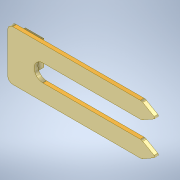
# Autodesk Inventor part: sensorhumedad
Saved by Autodesk Inventor 2022 (Build 260153000, 153)
## iProperties
Created: 2021-10-13
Part Number: sensorhumedad
Material: Brass, Soft Yellow
Document SubType Name: Modeling
Designer: pa.mahecha
Density: 8.47 g/cm^3
Appearance: Gold - Metal
Author: pa.mahecha
Autodesk Inventor part; units mm, degrees
ref_plane "YZ Plane" through (0, 0, 0) normal (1, 0, 0) x (0, 1, 0)
ref_plane "XZ Plane" through (0, 0, 0) normal (0, 1, 0) x (-1, 0, 0)
ref_plane "XY Plane" through (0, 0, 0) normal (0, 0, 1) x (1, 0, 0)
sketch "Sketch1" plane through (0, 0, 0) normal (0, 0, 1) x (1, 0, 0)
  line L0 (-9.4004, -0.0645) -> (24.8301, -0.0645)
  line L1 (-8.5062, -0.0645) -> (-8.5062, 8.0815)
  line L2 (-6.5062, 10.0815) -> (45.2045, 10.0815)
  line L3 (5.7396, 3.4575) -> (45.196, 3.4575)
  line L4 (-8.5062, -0.0645) -> (-8.5062, -8.2105)
  line L5 (-6.5062, -10.2105) -> (45.2045, -10.2105)
  line L6 (5.7396, -3.5865) -> (45.196, -3.5865)
  line L7 (50.7891, 7.186) -> (46.1991, 9.8167)
  line L8 (50.7862, 6.3168) -> (46.1793, 3.7159)
  line L9 (50.7891, -7.315) -> (46.1991, -9.9457)
  line L10 (50.7862, -6.4458) -> (46.1793, -3.8449)
  arc A0 (5.7396, 3.4575) -> (5.7396, -3.5865) centre (5.7054, -0.0645) ccw
  arc A1 (-6.5062, 10.0815) -> (-8.5062, 8.0815) centre (-6.5062, 8.0815) ccw
  arc A2 (-8.5062, -8.2105) -> (-6.5062, -10.2105) centre (-6.5062, -8.2105) ccw
  arc A3 (46.1991, 9.8167) -> (45.2045, 10.0815) centre (45.2045, 8.0815) ccw
  arc A4 (45.196, 3.4575) -> (46.1793, 3.7159) centre (45.196, 5.4575) ccw
  arc A5 (50.7862, 6.3168) -> (50.7891, 7.186) centre (50.5404, 6.7522) ccw
  line L11 (50.7891, -7.315) -> (46.1991, -9.9457)
  line L12 (50.7862, -6.4458) -> (46.1793, -3.8449)
  arc A6 (45.2045, -10.2105) -> (46.1991, -9.9457) centre (45.2045, -8.2105) ccw
  arc A7 (46.1793, -3.8449) -> (45.196, -3.5865) centre (45.196, -5.5865) ccw
  arc A8 (50.7891, -7.315) -> (50.7862, -6.4458) centre (50.5404, -6.8812) ccw
  line L13 (5.7396, 3.4575) -> (5.7396, 10.0815)
  line L14 (5.7396, -3.5865) -> (5.7396, -10.2105)
  point P0 (0, 0)
  point P1 (51.4938, 10.0604)
  point P2 (51.4938, -10.1894)
  dimension "d7" = 6.624
  dimension "d11" = 2
  dimension "d12" = 2
  dimension "d13" = 0.5
  constraints: 30 end point, 18 point on circle, 11 symmetric about line, 10 tangent, 9 centre point, 5 point on line, 2 equal radius, 2 horizontal, 2 perpendicular, 1 equal length, 1 vertical, 3 other
  measures "d7" distance between parallel lines of L3 L2
  measures "d11" radius of A1
  measures "d12" radius of A4
  measures "d13" radius of A5
extrude "Extrusion1" add sketch "Sketch1" along normal blind 1.5 contours L13 L2 A3 L7 A5 L8 A4 L3 | L6 A7 L10 A8 L9 A6 L5 L14
extrude "Extrusion2" add sketch "Sketch1" along normal blind 1.5 contours L1 A1 L2 L13 A0 L0 | L0 A0 L14 L5 A2 L4
split_face "Split1"
sketch "Sketch2" plane through (-8.5062, -8.2105, 0) normal (0, 0, -1) x (-1, 0, 0)
  line L0 (0, 16.292) -> (0, 0) projected
  line L1 (0, 13.3304) -> (-7.5479, 13.3304)
  line L2 (-7.5479, 13.3304) -> (-7.5479, 3.2425)
  line L3 (-7.5479, 3.2425) -> (0, 3.2425)
  line L4 (0, 3.2425) -> (0, 13.3304)
  line L5 (-8.5062, 8.2105) -> (18.1258, 8.2105)
  point P0 (0, 3.2425)
  dimension "d16" = 7.5479
  dimension "d17" = 10.0879
  dimension "d18" = 4.968
  constraints: 10 end point, 2 horizontal, 2 parallel, 1 perpendicular, 1 point on line
  measures "d16" distance of L2.end L3.end
  measures "d17" distance of L1.end L2.end
  measures "d18" distance from line of L5 L3.end
extrude "Extrusion3" add sketch "Sketch2" along normal blind 5.6
sketch "Sketch4" plane through (-8.5062, -8.2105, 1.5) normal (-1, 0, 0) x (0, 0, 1)
  line L0 (-1.5, 11.668) -> (-1.5, 18.292) projected
  line L1 (-6.093, 3.9575) -> (-1.5, 3.9575)
  line L2 (-1.5, 3.9575) -> (-1.5, 12.6111)
  line L3 (-1.5, 12.6111) -> (-6.093, 12.6111)
  line L4 (-7.1, 3.2425) -> (-7.1, 13.3304) projected
  line L5 (-1.5, 3.2425) -> (-7.1, 3.2425) projected
  line L6 (-1.5, 13.3304) -> (-7.1, 13.3304) projected
  line L7 (-1.5, 8.2105) -> (-9.0756, 8.2105)
  line L8 (-6.093, 6.97) -> (-6.5947, 6.97)
  line L9 (-6.5947, 6.97) -> (-6.5947, 8.2105)
  line L10 (-6.093, 9.4509) -> (-6.5947, 9.4509)
  line L11 (-6.5947, 9.4509) -> (-6.5947, 8.2105)
  line L12 (-6.093, 12.6111) -> (-6.093, 9.4509)
  line L13 (-6.093, 6.97) -> (-6.093, 3.9575)
  dimension "d22" = 0.715
  dimension "d23" = 0.7192
  constraints: 20 end point, 3 horizontal, 3 parallel, 2 perpendicular, 2 point on line, 2 symmetric about line
  measures "d22" distance between parallel lines of L1 L5
  measures "d23" distance between parallel lines of L6 L3
extrude "Extrusion4" cut sketch "Sketch4" against normal blind 7.4 contours L2 L7 L11 L10 L12 L3 L0 | L2 L1 L13 L8 L9 L7
body "Solid1"
